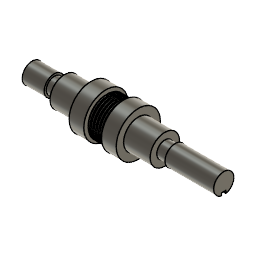
Roller 1 (Autodesk Fusion 360 design; units mm, degrees)
Autodesk Fusion 360 part; units mm, degrees
sketch "Sketch1" plane through (0, 0, 0) normal (1, 0, 0) x (0, 1, 0)
  circle A0 centre (0, 0) radius 10
  circle A1 centre (0, 0) radius 5.5
  circle A2 centre (0, 0) radius 6.9
  line L0 (-1.5, -6.735) -> (-1.5, -4.9)
  line L1 (-1.5, -4.9) -> (1.5, -4.9)
  line L2 (1.5, -4.9) -> (1.5, -6.735)
  line L3 (0, -11) -> (0, 11)
  line L4 (1.0311, 3.6) -> (1.4, 3.6)
  line L5 (1.4, 3.6) -> (1.4, 5.3188)
  line L6 (-1.0311, 3.6) -> (-1.4, 3.6)
  line L7 (-1.4, 3.6) -> (-1.4, 5.3188)
  line L8 (1.0311, 3.6) -> (-1.0311, 3.6)
  circle A3 centre (0, 0) radius 7.9
  circle A4 centre (0, 0) radius 15
  circle A5 centre (0, 0) radius 13
  circle A6 centre (0, 0) radius 12
  point P0 (0, -6.9)
  point P1 (0, 5.5)
  dimension "d1" = 20
  dimension "d4" = -4.5
  dimension "d11" = 13.8
  dimension "d15" = 3
  dimension "d16" = 2
  dimension "d31" = 2.8
  dimension "d32" = 1.9
  dimension "d55" = 1
  dimension "d56" = 5
  dimension "d57" = -2
  dimension "d58" = -1
  constraint coincident A0.centre A1.centre
  constraint coincident A2 L0.start
  constraint vertical L0
  constraint perpendicular L0 L1
  constraint coincident A2 L2.end
  constraint perpendicular L1 L2
  constraint vertical L3
  constraint symmetric L0 L2 L3
  constraint coincident A2 P0
  constraint coincident L3 P0
  constraint coincident A0.centre L3
  constraint horizontal L4
  constraint vertical L5
  constraint coincident A1 L5.end
  constraint horizontal L6
  constraint vertical L7
  constraint coincident A1 L7.end
  constraint perpendicular L3 L8
  constraint coincident L3 P1
  constraint coincident A1 P1
  constraint symmetric L3 L5 L7
  measures "d1" diameter of A0
  measures "d11" diameter of A2
  measures "d15" distance of L0 L2
  measures "d16" distance of L1 P0
  measures "d31" distance of L5 L7
  measures "d32" distance of L8 P1
extrude "Extrude1" add sketch "Sketch1" along normal blind 130 contours A0 L3 A3 | A0 L3 A3 | A2 L3 A3 | A2 L3 A3 | A1 A2 L0 L3 | A1 A2 L2 L3 | A1 A2 L2 L3 | A1 A2 L0 L3 | A1 L3 L6 L7 L8 | A1 L3 L4 L5 L8 | A1 L1 L2 L3 | A1 L0 L1 L3 | A1 L0 L1 L3 L6 L7 L8 | A1 L1 L2 L3 L4 L5 L8
extrude "Extrude2" cut sketch "Sketch1" along normal blind 7 from surface at 15 contours A0 L3 A3 | A0 L3 A3 | A2 L3 A3 | A2 L3 A3 | A1 A2 L0 L3 | A1 A2 L2 L3 | A1 A2 L2 L3 | A1 A2 L0 L3
extrude "Extrude3" cut sketch "Sketch1" along normal blind 7 from surface at 90 contours A0 L3 A3 | A0 L3 A3 | A2 L3 A3 | A2 L3 A3 | A1 A2 L0 L3 | A1 A2 L2 L3 | A1 A2 L2 L3 | A1 A2 L0 L3
extrude "Extrude4" cut sketch "Sketch1" along normal up to surface (33 mm away) from surface at 97 contours A0 L3 A3 | A0 L3 A3 | A2 L3 A3 | A2 L3 A3
extrude "Extrude5" cut sketch "Sketch1" along normal up to surface (24 mm away) from surface at 106 contours A1 A2 L2 L3 | A1 A2 L0 L3 | A1 L1 L2 L3 | A1 L0 L1 L3 picked at (0.8391, -5.9034) picked at (-0.8391, -5.9034)
extrude "Extrude6" cut sketch "Sketch1" along normal up to surface (15 mm away) contours A0 L3 A3 | A0 L3 A3 | A2 L3 A3 | A2 L3 A3
extrude "Extrude7" add sketch "Sketch1" along normal blind 32 from surface at 40 contours A4 | A5 | A6
extrude "Extrude8" cut sketch "Sketch1" along normal blind 10 contours A1 L1 L2 L3 | A1 L0 L1 L3 | A1 L0 L1 L3 L6 L7 L8 | A1 L1 L2 L3 L4 L5 L8
extrude "Extrude9" cut sketch "Sketch1" along normal blind 12 from surface at 50 contours A4
extrude "Extrude15" cut sketch "Sketch1" along normal blind 1 from surface at 50 contours A5
extrude "Extrude16" cut sketch "Sketch1" along normal blind 1 from surface at 52 contours A5
extrude "Extrude17" cut sketch "Sketch1" along normal blind 1 from surface at 54 contours A5
extrude "Extrude18" cut sketch "Sketch1" along normal blind 1 from surface at 56 contours A5
extrude "Extrude19" cut sketch "Sketch1" along normal blind 1 from surface at 58 contours A5
extrude "Extrude20" cut sketch "Sketch1" along normal blind 1 from surface at 60 contours A5
